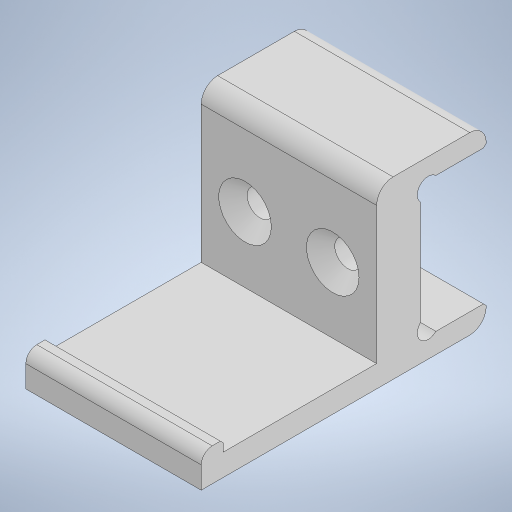
# Autodesk Inventor part: Door Bracket
Saved by Autodesk Inventor 2023.4 (Build 274418000, 418)
## iProperties
Created: 2024-08-27
Part Number: Door Bracket
Material: Generic
Document SubType Name: Modeling
Designer: Nathan Cai
Density: 1 g/cm^3
Appearance: Default
Author: Nathan Cai
Autodesk Inventor part; units mm, degrees
ref_plane "YZ Plane" through (0, 0, 0) normal (1, 0, 0) x (0, 1, 0)
ref_plane "XZ Plane" through (0, 0, 0) normal (0, 1, 0) x (-1, 0, 0)
ref_plane "XY Plane" through (0, 0, 0) normal (0, 0, 1) x (1, 0, 0)
sketch "Sketch1" plane through (0, 0, 0) normal (1, 0, 0) x (0, 1, 0)
  line L0 (-9.525, 4.7625) -> (9.525, 4.7625) construction
  line L1 (9.525, 4.7625) -> (9.525, -4.7625) construction
  line L2 (9.525, -4.7625) -> (-9.525, -4.7625) construction
  line L3 (-9.525, -4.7625) -> (-9.525, 4.7625) construction
  line L4 (-9.525, 4.7625) -> (9.525, -4.7625) construction
  line L5 (9.525, 4.7625) -> (-9.525, -4.7625) construction
  line L6 (-9.779, 4.7625) -> (9.779, 4.7625)
  line L7 (9.779, 4.7625) -> (9.779, -4.7625)
  line L8 (9.779, -4.7625) -> (-9.779, -4.7625) construction
  line L9 (-9.779, -4.7625) -> (-9.779, 4.7625)
  line L10 (-9.779, 4.7625) -> (9.779, -4.7625) construction
  line L11 (9.779, 4.7625) -> (-9.779, -4.7625) construction
  line L12 (-12.7, 11.1125) -> (12.7, 11.1125)
  line L13 (12.7, 11.1125) -> (12.7, -4.7625)
  line L14 (12.7, -4.7625) -> (-12.7, -4.7625)
  line L15 (-12.7, -4.7625) -> (-12.7, 11.1125)
  line L16 (-12.7, 11.1125) -> (12.7, -4.7625) construction
  line L17 (12.7, 11.1125) -> (-12.7, -4.7625) construction
  line L18 (0, 4.7625) -> (0, 0) construction
  line L19 (-12.7, 11.1125) -> (-9.525, 11.1125)
  line L20 (-9.525, 11.1125) -> (-9.525, 33.3375)
  line L21 (-9.525, 33.3375) -> (-12.7, 33.3375)
  line L22 (-12.7, 33.3375) -> (-12.7, 11.1125)
  line L23 (-12.7, 33.3375) -> (-9.525, 33.3375)
  line L24 (-9.525, 33.3375) -> (-9.525, 36.5125) construction
  line L25 (-9.525, 36.5125) -> (-12.7, 36.5125)
  line L26 (-12.7, 36.5125) -> (-12.7, 33.3375)
  circle A0 centre (-9.525, 34.925) radius 1.5875
  circle A1 centre (8.6565, 3.64) radius 1.5875
  line L27 (8.6565, 3.64) -> (9.779, 4.7625) construction
  circle A2 centre (-8.6565, 3.64) radius 1.5875
  line L28 (-9.525, 33.3375) -> (-7.9375, 33.3375)
  line L29 (-7.9375, 33.3375) -> (-7.9375, 34.925)
  line L30 (-7.9375, 34.925) -> (-9.525, 34.925) construction
  line L31 (-9.525, 34.925) -> (-9.525, 33.3375)
  point P0 (0, 3.175)
  point P1 (-9.525, 11.1125)
  point P2 (-9.525, 36.5125)
  point P3 (-9.779, 2.5174)
  point P4 (-7.5339, 4.7625)
  point P5 (7.5339, 4.7625)
  point P6 (9.779, 2.5174)
  dimension "d11" = 3.175
  dimension "d0" = 19.05
  dimension "d1" = 9.525
  dimension "d2" = 19.558
  dimension "d3" = 6.35
  dimension "d4" = 25.4
  dimension "d5" = 3.175
  dimension "d6" = 22.225
  dimension "d7" = 3.175
  dimension "d8" = 3.175
  constraints: 64 end point, 12 parallel, 8 midpoint, 6 horizontal, 6 perpendicular, 3 point on line, 2 centre point, 2 point on circle, 1 symmetric about line, 1 tangent, 1 vertical, 5 other
  measures "d0" distance of L1.end L2.end
  measures "d1" distance of L0.end L1.end
  measures "d2" distance between parallel lines of L9 L7
  measures "d3" distance between parallel lines of L0 L12
  measures "d4" distance between parallel lines of L15 L13
  measures "d5" distance of L21.end L20.end
  measures "d6" distance of L20.end L19.end
  measures "d7" distance of L25.end L24.end
  measures "d8" distance of L24.end L23.end
extrude "Extrusion1" add sketch "Sketch1" along normal blind 25.4 contours A2 L9 L14 L15 L12 L13 L7 A1 L6 | L22 L21 L20 L12 | L26 L25 A0 L21 | A0 | A0 L29 L28
chamfer "Chamfer1" distance 0.3969 angle 45 3 edges at (12.7, -9.779, -4.7625) (12.7, 9.779, -4.7625) (12.7, -7.9375, 33.3375)
fillet "Fillet1" radius 2.3813 2 edges at (12.7, 12.7, -4.7625) (12.7, -12.7, -4.7625)
fillet "Fillet2" radius 2.3813 1 edges at (12.7, 12.7, 11.1125)
sketch "Sketch2" plane through (0, -9.525, 11.1125) normal (0, 0, 1) x (1, 0, 0)
  line L0 (0, 19.8438) -> (0, 0) projected
  line L1 (0, 9.525) -> (25.4, 9.525) construction
  line L2 (25.4, 1.9911) -> (25.4, 17.0589) projected
  line L3 (25.4, 22.225) -> (0, 22.225) projected
  point P0 (0, 9.525)
  point P1 (6.35, 9.525)
  point P2 (19.05, 9.525)
  dimension "d17" = 12.7
  dimension "d18" = 6.35
  dimension "d21" = 12.7
  constraints: 2 end point, 2 horizontal, 2 point on line, 1 midpoint, 1 other
  measures "d17" distance between parallel lines of L3 L1
  measures "d18" distance from line of L0 point (6.35, 9.525)
  measures "d21" distance of point (6.35, 9.525) point (19.05, 9.525)
hole "Hole1" at (6.35, 0, 11.1125) at (19.05, 0, 11.1125) direction (0, 0, -1) diameter 3.81 end through all countersink diameter 7.62 countersink angle 82 clearance for "Flat Head Machine Screw (82)" size "#6" standard "Ansi Unified Screw Threads"
body "Solid1"
